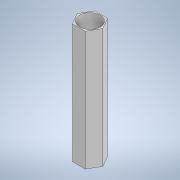
# Autodesk Inventor part: столбики
Saved by Autodesk Inventor 2021 (Build 250183000, 183)
## iProperties
Created: 2023-02-17
Part Number: столбики
Material: Типовые
Document SubType Name: Modeling
Designer: Tasya
Density: 1 g/cm^3
Appearance: По умолчанию
Author: Tasya
Autodesk Inventor part; units mm, degrees
ref_plane "YZ Plane" through (0, 0, 0) normal (1, 0, 0) x (0, 1, 0)
ref_plane "XZ Plane" through (0, 0, 0) normal (0, 1, 0) x (-1, 0, 0)
ref_plane "XY Plane" through (0, 0, 0) normal (0, 0, 1) x (1, 0, 0)
sketch "Эскиз1" plane through (0, 0, 0) normal (0, 1, 0) x (-1, 0, 0)
  circle A0 centre (0, 0) radius 1.4
  line L0 (0.8083, 1.4) -> (1.6166, 0)
  line L1 (1.6166, 0) -> (0.8083, -1.4)
  line L2 (0.8083, -1.4) -> (-0.8083, -1.4)
  line L3 (-0.8083, -1.4) -> (-1.6166, 0)
  line L4 (-1.6166, 0) -> (-0.8083, 1.4)
  line L5 (-0.8083, 1.4) -> (0.8083, 1.4)
  line L6 (0, 0) -> (3.2332, 0) construction
  dimension "d0" = 2.8
  constraints: 14 end point, 2 coincident, 1 centre point, 1 horizontal, 1 midpoint, 1 tangent, 13 other
  measures "d0" diameter of A0
extrude "Выдавливание1" add sketch "Эскиз1" along normal blind 15
sketch "Эскиз2" plane through (0, 15, 0) normal (0, 1, 0) x (1, 0, 0)
  point P0 (0, 0)
  point P1 (0, 0)
  constraints: 1 coincident
hole "Отверстие1" at (0, 15, 0) direction (0, -1, 0) diameter 2.6 depth 4
